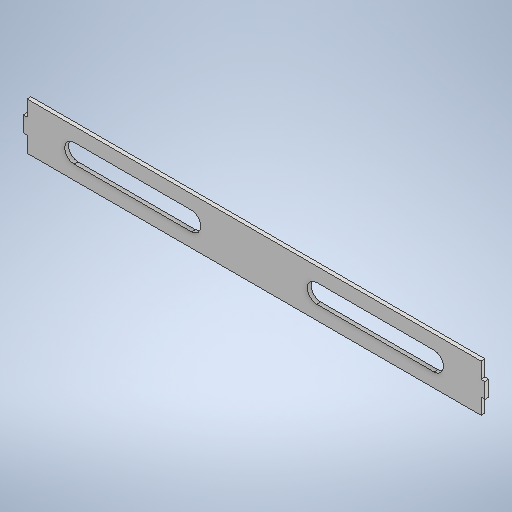
# Autodesk Inventor part: Table-Base Supporter 1st
Saved by Autodesk Inventor 2025.4 (Build 294407000, 407)
## iProperties
Created: 2026-05-09
Part Number: Table-Base Supporter 1st
Material: Generic
Document SubType Name: Sheet Metal
Designer: lenovo
Density: 1 g/cm^3
Sheet Metal Rule: Default_mm
Appearance: Default
Author: lenovo
Autodesk Inventor part; units mm, degrees
ref_plane "YZ Plane" through (0, 0, 0) normal (1, 0, 0) x (0, 1, 0)
ref_plane "XZ Plane" through (0, 0, 0) normal (0, 1, 0) x (-1, 0, 0)
ref_plane "XY Plane" through (0, 0, 0) normal (0, 0, 1) x (1, 0, 0)
sketch "Sketch1" plane through (0, 0, 0) normal (0, 0, 1) x (1, 0, 0)
  line L0 (-290, -30) -> (290, -30)
  line L1 (290, -30) -> (290, 30)
  line L2 (290, 30) -> (-290, 30)
  line L3 (-290, 30) -> (-290, -30)
  line L4 (-290, -30) -> (290, 30) construction
  line L5 (290, -30) -> (-290, 30) construction
  line L6 (-290, 9.925) -> (-294.9, 9.925)
  line L7 (-294.9, 9.925) -> (-294.9, -9.925)
  line L8 (-294.9, -9.925) -> (-290, -9.925)
  line L9 (-290, -9.925) -> (-290, 9.925)
  line L10 (0, 30) -> (0, -30)
  line L11 (290, 9.925) -> (294.9, 9.925)
  line L12 (294.9, 9.925) -> (294.9, -9.925)
  line L13 (294.9, -9.925) -> (290, -9.925)
  line L14 (290, -9.925) -> (290, 9.925)
  point P0 (0, 0)
  point P1 (-290, 0)
  point P2 (-290, 0)
  point P3 (290, 0)
  point P4 (290, 0)
  dimension "d0" = 580
  dimension "d1" = 60
  dimension "d2" = 4.9
  dimension "d3" = 19.85
  measures "d0" distance of L2.end L1.end
  measures "d1" distance of L1.end L0.end
  measures "d2" distance of L6.start L6.end
  measures "d3" distance of L6.end L7.end
extrude "Plate1" add sketch "Sketch1" along normal blind 5
sketch "Sketch2" plane through (0, 0, 5) normal (0, 0, 1) x (1, 0, 0)
  line L0 (-230, 0) -> (-80, 0) construction
  line L1 (-230, -12) -> (-80, -12)
  line L2 (-80, 12) -> (-230, 12)
  arc A0 (-230, 12) -> (-230, -12) centre (-230, 0) ccw
  arc A1 (-80, -12) -> (-80, 12) centre (-80, 0) ccw
  line L3 (0, 30) -> (0, -30)
  line L4 (290, -30) -> (-290, -30) projected
  line L5 (-290, 30) -> (290, 30) projected
  line L6 (230, 0) -> (80, 0) construction
  line L7 (230, -12) -> (80, -12)
  line L8 (80, 12) -> (230, 12)
  arc A2 (230, -12) -> (230, 12) centre (230, 0) ccw
  arc A3 (80, 12) -> (80, -12) centre (80, 0) ccw
  point P0 (0, 0)
  point P1 (-155, 0)
  point P2 (155, 0)
  dimension "d5" = 12
  dimension "d6" = 150
  dimension "d7" = 80
  constraints: 18 end point, 8 point on circle, 7 symmetric about line, 4 centre point, 4 tangent, 3 midpoint, 1 horizontal, 1 horizontal alignment, 1 parallel, 1 vertical, 2 other
  measures "d5" radius of A1
  measures "d6" distance of L0.start L0.end
  measures "d7" distance of point (0, 0) L0.end
extrude "Cut1" cut sketch "Sketch2" against normal blind 5
equation "\"d8\" = Thickness"
equation "\"d4\" = Thickness"
equation "\"BendRadius\" = Thickness"
equation "\"BendReliefWidth\" = Thickness"
equation "\"BendReliefDepth\" = 0.5 * Thickness"
equation "\"TransitionRadius\" = BendRadius"
equation "\"JacobiRadiusSize\" = BendRadius"
equation "\"GapSize\" = Thickness"
equation "\"Thickness\" = 5"
body "Solid1"
